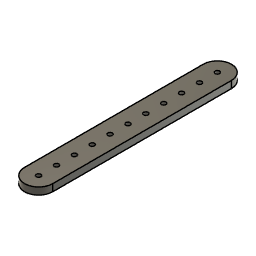
Camera arm 1 v5 (Autodesk Fusion 360 design; units mm, degrees)
Autodesk Fusion 360 part; units mm, degrees
sketch "Sketch1" plane through (0, 0, 0) normal (0, 1, 0) x (1, 0, 0)
  line L0 (20, 0) -> (20, -127)
  line L1 (0, -127) -> (0, 0)
  arc A0 (0, -127) -> (20, -127) centre (10, -127) ccw
  arc A1 (20, 0) -> (0, 0) centre (10, 0) ccw
  circle A2 centre (10, 0) radius 1.6
  circle A3 centre (10, -127) radius 1.6
  circle A4 centre (10, -114.3) radius 1.6
  circle A5 centre (10, -101.6) radius 1.6
  circle A6 centre (10, -88.9) radius 1.6
  circle A7 centre (10, -76.2) radius 1.6
  circle A8 centre (10, -63.5) radius 1.6
  circle A9 centre (10, -50.8) radius 1.6
  circle A10 centre (10, -38.1) radius 1.6
  circle A11 centre (10, -25.4) radius 1.6
  circle A12 centre (10, -12.7) radius 1.6
  dimension "d1" = 20
  dimension "d2" = 127
  dimension "d3" = 3.2
  dimension "d4" = 3.2
  dimension "d9" = 0
  dimension "d10" = 12.7
  constraint vertical L0
  constraint vertical L1
  constraint coincident L1.end A1.end
  constraint concentric A1 A2
  constraint concentric A0 A3
  measures "d1" distance of L1.end L0.start
  measures "d2" distance of L1.end L1.start
  measures "d3" diameter of A2
  measures "d4" diameter of A3
extrude "Extrude1" add sketch "Sketch1" along normal blind 5
